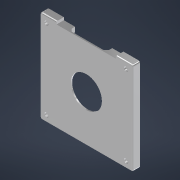
# Autodesk Inventor part: CUBIERTA DE SOPORTE BASE
Saved by Autodesk Inventor 2022 (Build 260153000, 153)
## iProperties
Created: 2021-09-22
Part Number: CUBIERTA DE SOPORTE BASE
Material: Aluminum 6061
Document SubType Name: Modeling
Designer: Andres
Density: 2.7 g/cm^3
Appearance: Aluminum - Flat
Author: Andres
Autodesk Inventor part; units mm, degrees
ref_plane "YZ Plane" through (0, 0, 0) normal (1, 0, 0) x (0, 1, 0)
ref_plane "XZ Plane" through (0, 0, 0) normal (0, 1, 0) x (-1, 0, 0)
ref_plane "XY Plane" through (0, 0, 0) normal (0, 0, 1) x (1, 0, 0)
sketch "Sketch1" plane through (0, 0, 0) normal (0, 0, 1) x (1, 0, 0)
  line L0 (-28, 58.66) -> (-28, 66) projected
  line L1 (-45, 70) -> (-67, 70) projected
  line L2 (-70, 67) -> (-70, -67) projected
  line L3 (-67, -70) -> (67, -70) projected
  line L4 (70, -67) -> (70, 67) projected
  line L5 (67, 70) -> (45, 70) projected
  line L6 (28, 66) -> (28, 58.66) projected
  arc A0 (-28, 58.66) -> (28, 58.66) centre (0, 0) ccw projected
  line L7 (-45, 66) -> (-45, 70) projected
  line L8 (45, 70) -> (45, 66) projected
  line L9 (45, 66) -> (28, 66) projected
  line L10 (-28, 66) -> (-45, 66) projected
  line L11 (28, 66) -> (-28, 66)
  circle A1 centre (-60, -60) radius 1.2295 projected
  circle A2 centre (60, 60) radius 1.2295 projected
  circle A3 centre (-60, 60) radius 1.2295 projected
  circle A4 centre (60, -60) radius 1.2295 projected
  arc A5 (70, 67) -> (67, 70) centre (67, 67) ccw projected
  arc A6 (-67, 70) -> (-70, 67) centre (-67, 67) ccw projected
  arc A7 (-70, -67) -> (-67, -70) centre (-67, -67) ccw projected
  arc A8 (67, -70) -> (70, -67) centre (67, -67) ccw projected
  constraints: 2 end point, 1 horizontal
extrude "Extrusion1" add sketch "Sketch1" along normal blind 9 contours A0 L6 L9 L8 L5 A5 L4 A8 L3 A7 L2 A6 L1 L7 L10 L0 | A1 | A2 | A3 | A4
sketch "Sketch2" plane through (0, 0, 9) normal (0, 0, 1) x (1, 0, 0)
  arc A0 (-28, 58.66) -> (28, 58.66) centre (0, 0) ccw projected
  line L0 (-28, 58.66) -> (-28, 66) projected
  line L1 (-28, 66) -> (-45, 66) projected
  line L2 (-45, 66) -> (-45, 70) projected
  line L3 (-45, 70) -> (-67, 70) projected
  line L4 (-70, 67) -> (-70, -67) projected
  line L5 (-67, -70) -> (67, -70) projected
  line L6 (70, -67) -> (70, 67) projected
  line L7 (67, 70) -> (45, 70) projected
  line L8 (45, 70) -> (45, 66) projected
  line L9 (45, 66) -> (28, 66) projected
  line L10 (28, 66) -> (28, 58.66) projected
  line L11 (28, 66) -> (28, 58.66) projected
  line L12 (-28, 58.66) -> (-28, 66) projected
  line L13 (28, 66) -> (-28, 66)
  circle A1 centre (0, 0) radius 22.5 projected
  circle A2 centre (0, 0) radius 23.5
  arc A3 (-67, 70) -> (-70, 67) centre (-67, 67) ccw projected
  arc A4 (-70, -67) -> (-67, -70) centre (-67, -67) ccw projected
  arc A5 (67, -70) -> (70, -67) centre (67, -67) ccw projected
  arc A6 (70, 67) -> (67, 70) centre (67, 67) ccw projected
  dimension "d4" = 1
  constraints: 2 end point, 1 centre point, 1 collinear
  measures "d4" radial gap between concentric circles of A1 A2
extrude "Extrusion2" add sketch "Sketch2" along normal blind 2 contours L0 L13 L10 A0 | A0 L10 L9 L8 L7 A6 L6 A5 L5 A4 L4 A3 L3 L2 L1 L0
sketch "Sketch3" plane through (0, 0, 11) normal (0, 0, 1) x (1, 0, 0)
  line L0 (-60, 60) -> (60, 60) construction
  line L1 (60, 60) -> (60, -60) construction
  line L2 (60, -60) -> (-60, -60) construction
  line L3 (-60, -60) -> (-60, 60) construction
  line L4 (-60, 60) -> (60, -60) construction
  line L5 (60, 60) -> (-60, -60) construction
  point P0 (0, 0)
  dimension "d5" = 120
  constraints: 12 end point, 4 coincident, 2 midpoint, 2 parallel, 2 perpendicular, 1 horizontal
  measures "d5" distance of L1.end L2.end
hole "Hole1" at (60, 60, 11) at (60, -60, 11) at (-60, -60, 11) at (-60, 60, 11) direction (0, 0, -1) diameter 3.4 end through all counterbore diameter 6.5 counterbore depth 3.4 clearance for "Socket Head Cap Screw ISO 4762" size "M3" standard "ISO"
chamfer "Chamfer1" distance 4 angle 45 3 edges at (0, -65, 9) (-28, 62.33, 9) (28, 62.33, 9)
fillet "Fillet1" radius 2 9 edges at (-69.1213, -69.1213, 11) (0, -70, 11) (69.1213, -69.1213, 11) (70, 0, 11) (69.1213, 69.1213, 11) (56, 70, 11) (-69.1213, 69.1213, 11) (-56, 70, 11) (-70, 0, 11)
body "Solid1"
